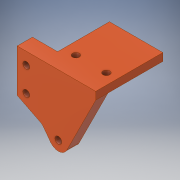
# Autodesk Inventor part: Hopper Idler
Saved by Autodesk Inventor 2018 (Build 220112000, 112)
## iProperties
Created: 2013-10-17
Part Number: Hopper Idler
Material: ABS Plastic
Document SubType Name: Modeling
Designer: Gabriel Smolnycki
Mass: 30.6616 g
Surface Area: 105.315 cm^2
Volume: 28.9261 cm^3
Density: 1.06 g/cm^3
Appearance: Smooth - Light Orange
Sending System: SolidWorks 2017
Last Author: Gabriel Smolnycki
Last Saved: 2017-09-14
Author: Gabriel Smolnycki
Autodesk Inventor part; units mm, degrees
note: some values were not read from the file. Chosen so that the rebuilt part matches the saved one: direction of "Hole5"; direction of "Hole4"; direction of "Hole3"; direction of "Hole2"; direction of "Hole1".
ref_plane "YZ Plane" through (0, 0, 0) normal (1, 0, 0) x (0, 1, 0)
ref_plane "XZ Plane" through (0, 0, 0) normal (0, 1, 0) x (-1, 0, 0)
ref_plane "XY Plane" through (0, 0, 0) normal (0, 0, 1) x (1, 0, 0)
sketch "Sketch1" plane through (0, 0, 0) normal (0, 0, 1) x (1, 0, 0)
  line L0 (-26.5, 28) -> (25, 28)
  line L1 (-26.5, 0) -> (-26.5, 28)
  line L2 (25, 28) -> (25, 23)
  arc A0 (-9.5, -9) -> (-10.9225, -7.8046) centre (-12.7143, -11.3809) ccw
  line L3 (-26.5, 0) -> (-10.9225, -7.8046)
  line L4 (-9.5, -9) -> (-4.5223, -15.7201)
  arc A1 (-4.5223, -15.7201) -> (6.0894, -14.7965) centre (0.5, -12) ccw
  line L5 (6.0894, -14.7965) -> (25, 23)
  constraints: 12 end point, 4 point on circle, 2 centre point, 2 vertical, 1 horizontal
extrude "Extrusion5" add sketch "Sketch1" against normal blind 44
sketch "Sketch2" plane through (0, 0, -44) normal (0, 0, -1) x (-1, 0, 0)
  line L0 (26.5, 0) -> (10.9225, -7.8046)
  arc A0 (-6.0894, -14.7965) -> (4.5223, -15.7201) centre (-0.5, -12) ccw
  line L1 (-25, 23) -> (0, 0)
  arc A1 (10.9225, -7.8046) -> (9.5, -9) centre (12.7143, -11.3809) ccw
  line L2 (-6.0894, -14.7965) -> (-25, 23)
  line L3 (0, 0) -> (26.5, 0)
  line L4 (9.5, -9) -> (4.5223, -15.7201)
  constraints: 10 end point, 4 point on circle, 2 centre point, 1 horizontal
extrude "Extrusion4" cut sketch "Sketch2" against normal blind 36
sketch "Sketch3" plane through (0, 0, -8) normal (0, 0, -1) x (-1, 0, 0)
  line L0 (0, 23) -> (0, 0)
  line L1 (-25, 23) -> (0, 23)
  line L2 (-25, 23) -> (0, 0)
  constraints: 6 end point, 1 horizontal, 1 vertical
extrude "Extrusion3" cut sketch "Sketch3" along normal blind 32
sketch "Sketch4" plane through (0, 0, -44) normal (0, 0, -1) x (-1, 0, 0)
  line L0 (10, 28) -> (10, 0)
  line L1 (10, 0) -> (26.5, 0)
  line L2 (10, 28) -> (26.5, 28)
  line L3 (26.5, 28) -> (26.5, 0)
  constraints: 8 end point, 2 horizontal, 2 vertical
extrude "Extrusion2" cut sketch "Sketch4" against normal blind 34 draft 0
hole "Hole6" at (-2, 28, -14) direction (0, -1, 0) diameter 4.5 depth 15
sketch "Sketch6" plane through (0, 23, -8) normal (0, -1, 0) x (1, 0, 0)
  line L0 (0, -2.5) -> (0, -4.9692)
  line L1 (-10, -9.5) -> (0, -9.5)
  line L2 (-10, -2.5) -> (0, -2.5)
  line L3 (0, -7.0308) -> (0, -9.5)
  arc A0 (0, -4.9692) -> (0, -7.0308) centre (-2, -6) ccw
  line L4 (-10, -2.5) -> (-10, -9.5)
  constraints: 10 end point, 3 vertical, 2 collinear, 2 horizontal, 2 point on circle, 1 centre point
extrude "Extrusion1" cut sketch "Sketch6" along normal blind 5
hole "Hole5" at (18, 28, -14) direction (0, -1, 0) diameter 4.5 depth 5
hole "Hole4" at (0, 17.5, -34) direction (-1, 0, 0) diameter 4.5 depth 10
sketch "Sketch8" plane through (0, 0, 0) normal (1, 0, 0) x (0, 1, 0)
  point P0 (17.5, -34)
hole "Hole3" at (0.5, -12, -8) direction (0, 0, 1) diameter 4.5 depth 8
sketch "Sketch7" plane through (-26.5, 28, 0) normal (0, 1, 0) x (1, 0, 0)
  point P0 (44.5, 14)
hole "Hole2" at (-20.5, 4, 0) direction (0, 0, -1) diameter 4.5 depth 10
sketch "Sketch5" plane through (-26.5, 28, 0) normal (0, 1, 0) x (1, 0, 0)
  point P0 (24.5, 14)
hole "Hole1" at (-20.5, 20, 0) direction (0, 0, -1) diameter 4.5 depth 10
sketch "Sketch9" plane through (0, 0, -8) normal (0, 0, -1) x (-1, 0, 0)
  point P0 (-0.5, -12)
sketch "Sketch10" plane through (0, 0, 0) normal (0, 0, 1) x (1, 0, 0)
  point P0 (-20.5, 4)
sketch "Sketch11" plane through (0, 0, 0) normal (0, 0, 1) x (1, 0, 0)
  point P0 (-20.5, 20)
body "Solid3"
